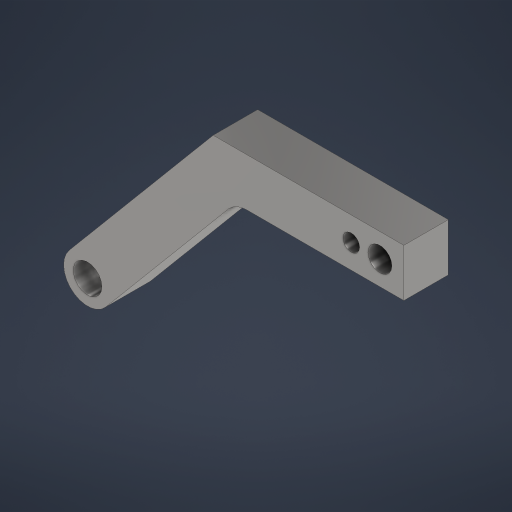
# Autodesk Inventor part: Servo_Strut_v2
Saved by Autodesk Inventor 2023 (Build 270158000, 158)
## iProperties
Created: 2023-02-25
Part Number: Servo_Strut_v2
Material: Steel, Carbon
Document SubType Name: Modeling
Designer: roota
Density: 7.85 g/cm^3
Appearance: Semi-Polished
Mass: 33.4264 g
Surface Area: 27.0753 cm^2
Volume: 4.25814 cm^3
Author: roota
Autodesk Inventor part; units mm, degrees
ref_plane "YZ Plane" through (0, 0, 0) normal (1, 0, 0) x (0, 1, 0)
ref_plane "XZ Plane" through (0, 0, 0) normal (0, 1, 0) x (-1, 0, 0)
ref_plane "XY Plane" through (0, 0, 0) normal (0, 0, 1) x (1, 0, 0)
sketch "Sketch1" plane through (0, 0, 0) normal (0, 0, 1) x (1, 0, 0)
  line L0 (0, 0) -> (-35.2056, 0)
  line L1 (-35.2056, 0) -> (-65.5234, -36.1314)
  line L2 (-65.5234, -36.1314) -> (-73.1839, -29.7035)
  line L3 (-73.1839, -29.7035) -> (-39.8687, 10)
  line L4 (-39.8687, 10) -> (0, 10)
  line L5 (0, 10) -> (0, 0)
  circle A0 centre (-66.1397, -29.0872) radius 3
  circle A1 centre (-5, 5) radius 2.5
  line L6 (0, 5) -> (-37.5371, 5) construction
  line L7 (-37.5371, 5) -> (-69.3536, -32.9174) construction
  line L8 (0, 0) -> (-65.5234, -36.1314) construction
  dimension "d0" = 10
  dimension "d1" = 6
  dimension "d2" = 5
  dimension "d3" = 5
  dimension "d4" = 5
  dimension "d5" = 70
  dimension "d26" = 50
  dimension "d28" = 17
  constraints: 18 end point, 3 perpendicular, 2 centre point, 2 horizontal, 2 midpoint, 2 parallel, 2 point on line, 1 equal length
  measures "d0" distance of L4.end L0.start
  measures "d1" diameter of A0
  measures "d2" diameter of A1
  measures "d3" distance from line of L5 A1.centre
  measures "d4" distance from line of L2 A0.centre
  measures "d5" distance of A1.centre A0.centre
  measures "d26" angle of L7 L0
  measures "d28" distance from line of L0.end L8
extrude "Extrusion1" add sketch "Sketch1" along normal blind 9.3
sketch "Sketch2" plane through (-73.1839, -29.7035, 9.3) normal (-0.7660444, 0.6427876, 0) x (0.6427876, 0.7660444, 0)
  line L0 (0, 9.3) -> (0, 0) projected
  line L1 (0, -5.7) -> (50, -5.7)
  line L2 (50, -5.7) -> (50, 4.3)
  line L3 (50, 4.3) -> (0, 4.3)
  line L4 (0, 4.3) -> (0, -5.7)
  point P0 (69.7959, 9.3)
  point P1 (0, 4.3)
  dimension "d10" = 5
  dimension "d11" = 10
  dimension "d13" = 50
  constraints: 8 end point, 2 parallel, 1 horizontal, 1 perpendicular, 1 point on line
  measures "d10" distance from line of L3 L0.start
  measures "d11" distance of L1.end L2.end
  measures "d13" distance of L1.start L1.end
extrude "Extrusion2" cut sketch "Sketch2" along normal blind 13
fillet "Fillet1" radius 5 5 edges at (-73.1839, -29.7035, 2.5) (-73.1823, -29.7048, 7.15) (-73.1831, -29.7041, 5) (-65.5234, -36.1314, 4.65) (-35.2056, 0, 4.65)
sketch "Sketch5" plane through (0, 0, 0) normal (0, 0, -1) x (-1, 0, 0)
  circle A0 centre (5, 5) radius 2.5 projected
  point P0 (0, 0)
  point P1 (11, 5)
  dimension "d29" = 6
  constraints: 1 horizontal alignment
  measures "d29" distance of A0.centre point (11, 5)
hole "Hole1" at (-11, 5, 0) direction (0, 0, 1) diameter 3.5 end through all
sketch "Sketch4" plane through (0, 0, 9.3) normal (0, 0, 1) x (1, 0, 0)
  line L0 (0, 0) -> (-30, 0)
  line L1 (-30, 0) -> (-30, 16.3827)
  line L2 (-30, 16.3827) -> (0, 16.3827)
  line L3 (0, 16.3827) -> (0, 0)
  dimension "d20" = 30
  constraints: 8 end point, 2 parallel, 1 coincident, 1 horizontal, 1 perpendicular
  measures "d20" distance of L1.end L2.end
equation "\"d3\" = 0.5 * d0"
equation "\"d4\" = 0.5 * d0"
body "Solid1"
